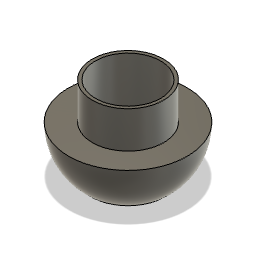
postreh_zarovka_v3 (Autodesk Fusion 360 design; units mm, degrees)
Autodesk Fusion 360 part; units mm, degrees
sketch "Sketch1" plane through (0, 0, 0) normal (0, 1, 0) x (1, 0, 0)
  circle A0 centre (0, 0) radius 25
  line L0 (23.097, 9.5671) -> (9.5671, 23.097)
  line L1 (9.5671, 23.097) -> (-9.5671, 23.097)
  line L2 (-9.5671, 23.097) -> (-23.097, 9.5671)
  line L3 (-23.097, 9.5671) -> (-23.097, -9.5671)
  line L4 (-23.097, -9.5671) -> (-9.5671, -23.097)
  line L5 (-9.5671, -23.097) -> (9.5671, -23.097)
  line L6 (9.5671, -23.097) -> (23.097, -9.5671)
  line L7 (23.097, -9.5671) -> (23.097, 9.5671)
  circle A1 centre (0, 0) radius 14
  line L8 (-5.25, 23.497) -> (5.25, 23.497)
  line L9 (5.25, 23.497) -> (5.25, 22.697)
  line L10 (5.25, 22.697) -> (-5.25, 22.697)
  line L11 (-5.25, 22.697) -> (-5.25, 23.497)
  line L12 (-5.25, 23.497) -> (5.25, 22.697) construction
  line L13 (5.25, 23.497) -> (-5.25, 22.697) construction
  line L14 (4.25, 25.2724) -> (-4.25, 25.2724)
  line L15 (-4.25, 25.2724) -> (-4.25, 21.7216)
  line L16 (-4.25, 21.7216) -> (4.25, 21.7216)
  line L17 (4.25, 21.7216) -> (4.25, 25.2724)
  line L18 (4.25, 25.2724) -> (-4.25, 21.7216) construction
  line L19 (-4.25, 25.2724) -> (4.25, 21.7216) construction
  line L20 (-12.3369, 19.7615) -> (-19.7615, 12.3369)
  line L21 (-12.9026, 20.3272) -> (-12.3369, 19.7615)
  line L22 (-20.3272, 12.9026) -> (-12.9026, 20.3272)
  line L23 (-12.3543, 18.3647) -> (-14.8651, 20.8755)
  line L24 (-18.3647, 12.3543) -> (-12.3543, 18.3647)
  line L25 (-20.8755, 14.8651) -> (-18.3647, 12.3543)
  line L26 (-19.7615, 12.3369) -> (-20.3272, 12.9026)
  line L27 (-14.8651, 20.8755) -> (-20.8755, 14.8651)
  line L28 (-22.697, 5.25) -> (-22.697, -5.25)
  line L29 (-23.497, 5.25) -> (-22.697, 5.25)
  line L30 (-23.497, -5.25) -> (-23.497, 5.25)
  line L31 (-21.7216, 4.25) -> (-25.2724, 4.25)
  line L32 (-21.7216, -4.25) -> (-21.7216, 4.25)
  line L33 (-25.2724, -4.25) -> (-21.7216, -4.25)
  line L34 (-22.697, -5.25) -> (-23.497, -5.25)
  line L35 (-25.2724, 4.25) -> (-25.2724, -4.25)
  line L36 (-19.7615, -12.3369) -> (-12.3369, -19.7615)
  line L37 (-20.3272, -12.9026) -> (-19.7615, -12.3369)
  line L38 (-12.9026, -20.3272) -> (-20.3272, -12.9026)
  line L39 (-18.3647, -12.3543) -> (-20.8755, -14.8651)
  line L40 (-12.3543, -18.3647) -> (-18.3647, -12.3543)
  line L41 (-14.8651, -20.8755) -> (-12.3543, -18.3647)
  line L42 (-12.3369, -19.7615) -> (-12.9026, -20.3272)
  line L43 (-20.8755, -14.8651) -> (-14.8651, -20.8755)
  line L44 (-5.25, -22.697) -> (5.25, -22.697)
  line L45 (-5.25, -23.497) -> (-5.25, -22.697)
  line L46 (5.25, -23.497) -> (-5.25, -23.497)
  line L47 (-4.25, -21.7216) -> (-4.25, -25.2724)
  line L48 (4.25, -21.7216) -> (-4.25, -21.7216)
  line L49 (4.25, -25.2724) -> (4.25, -21.7216)
  line L50 (5.25, -22.697) -> (5.25, -23.497)
  line L51 (-4.25, -25.2724) -> (4.25, -25.2724)
  line L52 (12.3369, -19.7615) -> (19.7615, -12.3369)
  line L53 (12.9026, -20.3272) -> (12.3369, -19.7615)
  line L54 (20.3272, -12.9026) -> (12.9026, -20.3272)
  line L55 (12.3543, -18.3647) -> (14.8651, -20.8755)
  line L56 (18.3647, -12.3543) -> (12.3543, -18.3647)
  line L57 (20.8755, -14.8651) -> (18.3647, -12.3543)
  line L58 (19.7615, -12.3369) -> (20.3272, -12.9026)
  line L59 (14.8651, -20.8755) -> (20.8755, -14.8651)
  line L60 (22.697, -5.25) -> (22.697, 5.25)
  line L61 (23.497, -5.25) -> (22.697, -5.25)
  line L62 (23.497, 5.25) -> (23.497, -5.25)
  line L63 (21.7216, -4.25) -> (25.2724, -4.25)
  line L64 (21.7216, 4.25) -> (21.7216, -4.25)
  line L65 (25.2724, 4.25) -> (21.7216, 4.25)
  line L66 (22.697, 5.25) -> (23.497, 5.25)
  line L67 (25.2724, -4.25) -> (25.2724, 4.25)
  line L68 (19.7615, 12.3369) -> (12.3369, 19.7615)
  line L69 (20.3272, 12.9026) -> (19.7615, 12.3369)
  line L70 (12.9026, 20.3272) -> (20.3272, 12.9026)
  line L71 (18.3647, 12.3543) -> (20.8755, 14.8651)
  line L72 (12.3543, 18.3647) -> (18.3647, 12.3543)
  line L73 (14.8651, 20.8755) -> (12.3543, 18.3647)
  line L74 (12.3369, 19.7615) -> (12.9026, 20.3272)
  line L75 (20.8755, 14.8651) -> (14.8651, 20.8755)
  point P0 (0, 23.097)
  point P1 (0, 23.497)
  dimension "d1" = 50
  dimension "d2" = 28
  dimension "d3" = 10.5
  dimension "d4" = 0.8
  dimension "d5" = 8.5
  dimension "d7" = 360
  constraint coincident A0.centre A1.centre
  constraint coincident A0 L0.start
  constraint concentric A0 A1
  constraint horizontal L8
  constraint perpendicular L8 L9
  constraint parallel L8 L10
  constraint parallel L9 L11
  constraint coincident L12 P0
  constraint coincident L13 P0
  constraint midpoint L1 P0
  constraint horizontal L14
  constraint perpendicular L14 L15
  constraint parallel L14 L16
  constraint parallel L15 L17
  constraint coincident L18 P1
  constraint coincident L19 P1
  constraint midpoint L8 P1
  measures "d1" diameter of A0
  measures "d2" diameter of A1
  measures "d3" distance of L9.end L10.end
  measures "d4" distance of L8.end L9.end
  measures "d5" distance of L15.end L16.end
extrude "Extrude1" add sketch "Sketch1" along normal blind 105 contours A0 L7 L62 L65 L66 | A0 L7 L61 L62 L63 | A0 L0 L69 L70 L71 | L0 L1 L2 L3 L4 L5 L6 L7 L9 L10 L11 L15 L16 L17 L20 L21 L23 L24 L25 L26 L28 L29 L31 L32 L33 L34 L36 L37 L39 L40 L41 L42 L44 L45 L47 L48 L49 L50 L52 L53 L55 L56 L57 L58 L60 L61 L63 L64 L65 L66 L68 L69 L71 L72 L73 L74 | A0 L6 L54 L57 L58 | A0 L0 L70 L73 L74 | L60 L63 L64 L65 | A0 L6 L53 L54 L55 | A0 L1 L8 L9 L17 | L68 L71 L72 L73 | A0 L5 L46 L49 L50 | L52 L55 L56 L57 | A0 L1 L8 L11 L15 | A0 L5 L45 L46 L47 | A0 L2 L21 L22 L23 | L10 L15 L16 L17 | A0 L4 L38 L41 L42 | L44 L47 L48 L49 | A0 L2 L22 L25 L26 | A0 L4 L37 L38 L39 | A0 L3 L29 L30 L31 | L20 L23 L24 L25 | A0 L3 L30 L33 L34 | L36 L39 L40 L41 | L28 L31 L32 L33 makes body 1
sketch "Sketch2" plane through (0, 0, 0) normal (0, 1, 0) x (1, 0, 0)
  circle A0 centre (91.4073, -5.9758) radius 17.5
  circle A1 centre (75.1447, -64.4139) radius 16.25
  dimension "d10" = 35
  dimension "d11" = 32.5
  measures "d10" diameter of A0
  measures "d11" diameter of A1
sketch "Sketch3" plane through (0, 105, 0) normal (0, 1, 0) x (-1, 0, 0)
  circle A0 centre (0, 0) radius 14
  line L0 (-19.6201, -13.6097) -> (-20.3272, -12.9026)
  line L1 (-20.3272, -12.9026) -> (-19.7615, -12.3369)
  line L2 (-19.7615, -12.3369) -> (-12.3369, -19.7615)
  line L3 (-12.3369, -19.7615) -> (-12.9026, -20.3272)
  line L4 (-12.9026, -20.3272) -> (-13.6097, -19.6201)
  line L5 (-13.6097, -19.6201) -> (-14.4152, -20.4256)
  arc A1 (-14.4152, -20.4256) -> (-4.25, -24.6361) centre (0, 0) ccw
  line L6 (-4.25, -24.6361) -> (-4.25, -23.497)
  line L7 (-4.25, -23.497) -> (-5.25, -23.497)
  line L8 (-5.25, -23.497) -> (-5.25, -22.697)
  line L9 (-5.25, -22.697) -> (5.25, -22.697)
  line L10 (5.25, -22.697) -> (5.25, -23.497)
  line L11 (5.25, -23.497) -> (4.25, -23.497)
  line L12 (4.25, -23.497) -> (4.25, -24.6361)
  arc A2 (4.25, -24.6361) -> (14.4152, -20.4256) centre (0, 0) ccw
  line L13 (14.4152, -20.4256) -> (13.6097, -19.6201)
  line L14 (13.6097, -19.6201) -> (12.9026, -20.3272)
  line L15 (12.9026, -20.3272) -> (12.3369, -19.7615)
  line L16 (12.3369, -19.7615) -> (19.7615, -12.3369)
  line L17 (19.7615, -12.3369) -> (20.3272, -12.9026)
  line L18 (20.3272, -12.9026) -> (19.6201, -13.6097)
  line L19 (19.6201, -13.6097) -> (20.4256, -14.4152)
  arc A3 (20.4256, -14.4152) -> (24.6361, -4.25) centre (0, 0) ccw
  line L20 (24.6361, -4.25) -> (23.497, -4.25)
  line L21 (23.497, -4.25) -> (23.497, -5.25)
  line L22 (23.497, -5.25) -> (22.697, -5.25)
  line L23 (22.697, -5.25) -> (22.697, 5.25)
  line L24 (22.697, 5.25) -> (23.497, 5.25)
  line L25 (23.497, 5.25) -> (23.497, 4.25)
  line L26 (23.497, 4.25) -> (24.6361, 4.25)
  arc A4 (24.6361, 4.25) -> (20.4256, 14.4152) centre (0, 0) ccw
  line L27 (20.4256, 14.4152) -> (19.6201, 13.6097)
  line L28 (19.6201, 13.6097) -> (20.3272, 12.9026)
  line L29 (20.3272, 12.9026) -> (19.7615, 12.3369)
  line L30 (19.7615, 12.3369) -> (12.3369, 19.7615)
  line L31 (12.3369, 19.7615) -> (12.9026, 20.3272)
  line L32 (12.9026, 20.3272) -> (13.6097, 19.6201)
  line L33 (13.6097, 19.6201) -> (14.4152, 20.4256)
  arc A5 (14.4152, 20.4256) -> (4.25, 24.6361) centre (0, 0) ccw
  line L34 (4.25, 24.6361) -> (4.25, 23.497)
  line L35 (4.25, 23.497) -> (5.25, 23.497)
  line L36 (5.25, 23.497) -> (5.25, 22.697)
  line L37 (5.25, 22.697) -> (-5.25, 22.697)
  line L38 (-5.25, 22.697) -> (-5.25, 23.497)
  line L39 (-5.25, 23.497) -> (-4.25, 23.497)
  line L40 (-4.25, 23.497) -> (-4.25, 24.6361)
  arc A6 (-4.25, 24.6361) -> (-14.4152, 20.4256) centre (0, 0) ccw
  line L41 (-14.4152, 20.4256) -> (-13.6097, 19.6201)
  line L42 (-13.6097, 19.6201) -> (-12.9026, 20.3272)
  line L43 (-12.9026, 20.3272) -> (-12.3369, 19.7615)
  line L44 (-12.3369, 19.7615) -> (-19.7615, 12.3369)
  line L45 (-19.7615, 12.3369) -> (-20.3272, 12.9026)
  line L46 (-20.3272, 12.9026) -> (-19.6201, 13.6097)
  line L47 (-19.6201, 13.6097) -> (-20.4256, 14.4152)
  arc A7 (-20.4256, 14.4152) -> (-24.6361, 4.25) centre (0, 0) ccw
  line L48 (-24.6361, 4.25) -> (-23.497, 4.25)
  line L49 (-23.497, 4.25) -> (-23.497, 5.25)
  line L50 (-23.497, 5.25) -> (-22.697, 5.25)
  line L51 (-22.697, 5.25) -> (-22.697, -5.25)
  line L52 (-22.697, -5.25) -> (-23.497, -5.25)
  line L53 (-23.497, -5.25) -> (-23.497, -4.25)
  line L54 (-23.497, -4.25) -> (-24.6361, -4.25)
  arc A8 (-24.6361, -4.25) -> (-20.4256, -14.4152) centre (0, 0) ccw
  line L55 (-20.4256, -14.4152) -> (-19.6201, -13.6097)
  circle A9 centre (0, 0) radius 17.5
  dimension "d16" = 35
  constraint concentric A0 A9
  measures "d16" diameter of A9
extrude "Extrude3" add sketch "Sketch3" along normal blind 12 contours A0 | A9 bodies 1
chamfer "Chamfer1" distance 4 angle 45 1 edges at (-13.0526, 105, -5.0626) on bodies 1
extrude "Extrude4" cut 1 faces at (-2.8212, 105, -0.9825) along direction (0, 1, 0) blind 44 on bodies 1 bodies 1
ref_plane "WorkPlane3" through (0, 117, 0) normal (0, 1, 0) x (-1, 0, 0)
ref_plane "WorkPlane4" through (0, 114, 0) normal (0, 1, 0) x (-1, 0, 0)
ref_plane "WorkPlane5" through (0, 111, 0) normal (0, 1, 0) x (-1, 0, 0)
thread "Thread3" "ANSI Unified Screw Threads 1.375 1 3/8-8 UN 3A" major diameter 34.7345 minor diameter 31.1455 pitch 3.175 angle 60 modelled right hand crest width 0.4671 on face at (-17.4433, 113, -1.4082) crest through (-17.3672, 104.2062, 0) on bodies 1
sketch "Sketch4" plane through (0, 105, 0) normal (0, 1, 0) x (-1, 0, 0)
  arc A0 (7.7444, 15.545) -> (-7.7444, 15.545) centre (0, 0) ccw
  spline S0 degree 3 poles (7.7444, 15.545) (8.9942, 14.8417) (10.1519, 13.9862) (12.214, 12.0191) (13.1134, 10.9184) (15.0227, 7.8711) (15.8119, 5.8174) (16.5433, 1.5647) (16.4948, -0.5901) (15.5763, -4.7155) (14.7314, -6.6497) (12.3661, -10.0449) (10.8824, -11.4824) (9.1629, -12.5917) knots -3.386882 -3.386882 -3.386882 -3.386882 -2.957534 -2.957534 -2.533537 -2.533537 -1.880654 -1.880654 -1.240767 -1.240767 -0.613881 -0.613881 0 0 0 0
  arc A1 (-9.1629, -12.5917) -> (9.1629, -12.5917) centre (0, 0) ccw
  spline S1 degree 3 poles (-9.1629, -12.5917) (-10.2571, -11.8858) (-11.2583, -11.0453) (-13.0433, -9.1242) (-13.8169, -8.0481) (-15.4568, -5.0428) (-16.0901, -3.016) (-16.5572, 1.21) (-16.3698, 3.3701) (-15.173, 7.5422) (-14.1591, 9.5092) (-11.4129, 12.984) (-9.6941, 14.4478) (-7.7444, 15.545) knots -3.394641 -3.394641 -3.394641 -3.394641 -3.003225 -3.003225 -2.606447 -2.606447 -1.974373 -1.974373 -1.32927 -1.32927 -0.671144 -0.671144 0 0 0 0
  line L0 (-19.6201, -13.6097) -> (-20.3272, -12.9026)
  line L1 (-20.3272, -12.9026) -> (-19.7615, -12.3369)
  line L2 (-19.7615, -12.3369) -> (-12.3369, -19.7615)
  line L3 (-12.3369, -19.7615) -> (-12.9026, -20.3272)
  line L4 (-12.9026, -20.3272) -> (-13.6097, -19.6201)
  line L5 (-13.6097, -19.6201) -> (-14.4152, -20.4256)
  arc A2 (-14.4152, -20.4256) -> (-4.25, -24.6361) centre (0, 0) ccw
  line L6 (-4.25, -24.6361) -> (-4.25, -23.497)
  line L7 (-4.25, -23.497) -> (-5.25, -23.497)
  line L8 (-5.25, -23.497) -> (-5.25, -22.697)
  line L9 (-5.25, -22.697) -> (5.25, -22.697)
  line L10 (5.25, -22.697) -> (5.25, -23.497)
  line L11 (5.25, -23.497) -> (4.25, -23.497)
  line L12 (4.25, -23.497) -> (4.25, -24.6361)
  arc A3 (4.25, -24.6361) -> (14.4152, -20.4256) centre (0, 0) ccw
  line L13 (14.4152, -20.4256) -> (13.6097, -19.6201)
  line L14 (13.6097, -19.6201) -> (12.9026, -20.3272)
  line L15 (12.9026, -20.3272) -> (12.3369, -19.7615)
  line L16 (12.3369, -19.7615) -> (19.7615, -12.3369)
  line L17 (19.7615, -12.3369) -> (20.3272, -12.9026)
  line L18 (20.3272, -12.9026) -> (19.6201, -13.6097)
  line L19 (19.6201, -13.6097) -> (20.4256, -14.4152)
  arc A4 (20.4256, -14.4152) -> (24.6361, -4.25) centre (0, 0) ccw
  line L20 (24.6361, -4.25) -> (23.497, -4.25)
  line L21 (23.497, -4.25) -> (23.497, -5.25)
  line L22 (23.497, -5.25) -> (22.697, -5.25)
  line L23 (22.697, -5.25) -> (22.697, 5.25)
  line L24 (22.697, 5.25) -> (23.497, 5.25)
  line L25 (23.497, 5.25) -> (23.497, 4.25)
  line L26 (23.497, 4.25) -> (24.6361, 4.25)
  arc A5 (24.6361, 4.25) -> (20.4256, 14.4152) centre (0, 0) ccw
  line L27 (20.4256, 14.4152) -> (19.6201, 13.6097)
  line L28 (19.6201, 13.6097) -> (20.3272, 12.9026)
  line L29 (20.3272, 12.9026) -> (19.7615, 12.3369)
  line L30 (19.7615, 12.3369) -> (12.3369, 19.7615)
  line L31 (12.3369, 19.7615) -> (12.9026, 20.3272)
  line L32 (12.9026, 20.3272) -> (13.6097, 19.6201)
  line L33 (13.6097, 19.6201) -> (14.4152, 20.4256)
  arc A6 (14.4152, 20.4256) -> (4.25, 24.6361) centre (0, 0) ccw
  line L34 (4.25, 24.6361) -> (4.25, 23.497)
  line L35 (4.25, 23.497) -> (5.25, 23.497)
  line L36 (5.25, 23.497) -> (5.25, 22.697)
  line L37 (5.25, 22.697) -> (-5.25, 22.697)
  line L38 (-5.25, 22.697) -> (-5.25, 23.497)
  line L39 (-5.25, 23.497) -> (-4.25, 23.497)
  line L40 (-4.25, 23.497) -> (-4.25, 24.6361)
  arc A7 (-4.25, 24.6361) -> (-14.4152, 20.4256) centre (0, 0) ccw
  line L41 (-14.4152, 20.4256) -> (-13.6097, 19.6201)
  line L42 (-13.6097, 19.6201) -> (-12.9026, 20.3272)
  line L43 (-12.9026, 20.3272) -> (-12.3369, 19.7615)
  line L44 (-12.3369, 19.7615) -> (-19.7615, 12.3369)
  line L45 (-19.7615, 12.3369) -> (-20.3272, 12.9026)
  line L46 (-20.3272, 12.9026) -> (-19.6201, 13.6097)
  line L47 (-19.6201, 13.6097) -> (-20.4256, 14.4152)
  arc A8 (-20.4256, 14.4152) -> (-24.6361, 4.25) centre (0, 0) ccw
  line L48 (-24.6361, 4.25) -> (-23.497, 4.25)
  line L49 (-23.497, 4.25) -> (-23.497, 5.25)
  line L50 (-23.497, 5.25) -> (-22.697, 5.25)
  line L51 (-22.697, 5.25) -> (-22.697, -5.25)
  line L52 (-22.697, -5.25) -> (-23.497, -5.25)
  line L53 (-23.497, -5.25) -> (-23.497, -4.25)
  line L54 (-23.497, -4.25) -> (-24.6361, -4.25)
  arc A9 (-24.6361, -4.25) -> (-20.4256, -14.4152) centre (0, 0) ccw
  line L55 (-20.4256, -14.4152) -> (-19.6201, -13.6097)
  circle A10 centre (0, 0) radius 27.4518
  circle A11 centre (0, 0) radius 18
  line L56 (19.7615, -12.3369) -> (12.3369, -19.7615)
  line L57 (5.25, -22.697) -> (12.3369, -19.7615)
  line L58 (5.25, -22.697) -> (-5.25, -22.697)
  line L59 (-5.25, -22.697) -> (-12.3369, -19.7615)
  line L60 (-19.7615, -12.3369) -> (-12.3369, -19.7615)
  line L61 (-19.7615, -12.3369) -> (-22.697, -5.25)
  line L62 (-22.697, -5.25) -> (-22.697, 5.25)
  line L63 (-22.697, 5.25) -> (-19.7615, 12.3369)
  line L64 (-19.7615, 12.3369) -> (-12.3369, 19.7615)
  line L65 (-12.3369, 19.7615) -> (-5.25, 22.697)
  line L66 (-5.25, 22.697) -> (5.25, 22.697)
  line L67 (5.25, 22.697) -> (12.3369, 19.7615)
  line L68 (12.3369, 19.7615) -> (19.7615, 12.3369)
  line L69 (19.7615, 12.3369) -> (22.697, 5.25)
  line L70 (22.697, 5.25) -> (22.697, -5.25)
  line L71 (22.697, -5.25) -> (19.7615, -12.3369)
  dimension "d25" = 36
  constraint concentric A0 A10
  constraint concentric A0 A11
  constraint coincident L16.end L17.start
  constraint coincident L15.end L16.start
  constraint coincident L9.end L10.start
  constraint coincident L8.end L9.start
  constraint coincident L2.end L3.start
  constraint coincident L1.end L2.start
  constraint coincident L51.end L52.start
  constraint coincident L50.end L51.start
  constraint coincident L44.end L45.start
  constraint coincident L43.end L44.start
  constraint coincident L37.end L38.start
  constraint coincident L36.end L37.start
  constraint coincident L30.end L31.start
  constraint coincident L29.end L30.start
  constraint coincident L23.end L24.start
  constraint coincident L22.end L23.start
  measures "d25" diameter of A11
extrude "Extrude5" cut sketch "Sketch4" against normal blind 8 contours L0 L1 L52 L53 L54 A9 L55 L61 | L3 L4 L5 A2 L6 L7 L8 L59 | L45 L46 L47 A8 L48 L49 L50 L63 | L10 L11 L12 A3 L13 L14 L15 L57 | L38 L39 L40 A7 L41 L42 L43 L65 | L17 L18 L19 A4 L20 L21 L22 L71 | L31 L32 L33 A6 L34 L35 L36 L67 | L24 L25 L26 A5 L27 L28 L29 L69 bodies 1
sketch "Sketch5" plane through (21.2292, 0, 8.7934) normal (0.92388, 0, 0.382683) x (0.382683, 0, -0.92388)
  line L0 (3.8354, 105) -> (-3.8354, 105)
  line L1 (-3.8354, 105) -> (-3.8354, 97)
  line L2 (-3.8354, 97) -> (3.8354, 97)
  line L3 (3.8354, 97) -> (3.8354, 105)
  line L4 (-3.8354, 105) -> (3.8354, 105)
  line L5 (3.8354, 105) -> (3.8354, 97.329)
  line L6 (3.8354, 97.329) -> (-3.8354, 97.329)
  line L7 (-3.8354, 97.329) -> (-3.8354, 105)
  circle A0 centre (0, 101) radius 2.5
  dimension "d28" = 7.671
  dimension "d29" = 5
  constraint horizontal L4
  constraint vertical L5
  constraint horizontal L6
  constraint vertical L7
  constraint coincident L0.end L1.start
  measures "d28" distance of L0.end L6.end
  measures "d29" diameter of A0
extrude "Extrude6" cut sketch "Sketch5" against normal blind 52 contours A0 bodies 1
sketch "Sketch6" plane through (21.2292, 0, -8.7934) normal (0.92388, 0, -0.382683) x (-0.382683, 0, -0.92388)
  line L0 (3.8354, 105) -> (-3.8354, 105)
  line L1 (-3.8354, 105) -> (-3.8354, 97)
  line L2 (-3.8354, 97) -> (3.8354, 97)
  line L3 (3.8354, 97) -> (3.8354, 105)
  line L4 (-3.8354, 105) -> (3.8354, 105)
  line L5 (3.8354, 105) -> (3.8354, 97.329)
  line L6 (3.8354, 97.329) -> (-3.8354, 97.329)
  line L7 (-3.8354, 97.329) -> (-3.8354, 105)
  circle A0 centre (0, 101.1645) radius 2.5
  dimension "d32" = 7.671
  dimension "d33" = 5
  constraint horizontal L4
  constraint vertical L5
  constraint horizontal L6
  constraint vertical L7
  constraint coincident L0.end L1.start
  measures "d32" distance of L0.end L6.end
  measures "d33" diameter of A0
extrude "Extrude7" cut sketch "Sketch6" against normal blind 103 contours A0 bodies 1
sketch "Sketch7" plane through (8.7934, 0, -21.2292) normal (0.382683, 0, -0.92388) x (-0.92388, 0, -0.382683)
  line L0 (3.8354, 105) -> (-3.8354, 105)
  line L1 (-3.8354, 105) -> (-3.8354, 97)
  line L2 (-3.8354, 97) -> (3.8354, 97)
  line L3 (3.8354, 97) -> (3.8354, 105)
  line L4 (-3.8354, 105) -> (3.8354, 105)
  line L5 (3.8354, 105) -> (3.8354, 97.329)
  line L6 (3.8354, 97.329) -> (-3.8354, 97.329)
  line L7 (-3.8354, 97.329) -> (-3.8354, 105)
  circle A0 centre (0, 101) radius 2.5
  dimension "d36" = 7.671
  dimension "d37" = 5
  constraint horizontal L4
  constraint vertical L5
  constraint horizontal L6
  constraint vertical L7
  constraint coincident L0.end L1.start
  measures "d36" distance of L0.end L6.end
  measures "d37" diameter of A0
extrude "Extrude8" cut sketch "Sketch7" against normal blind 84 contours A0 bodies 1
sketch "Sketch8" plane through (-8.7934, 0, -21.2292) normal (-0.382683, 0, -0.92388) x (-0.92388, 0, 0.382683)
  line L0 (3.8354, 105) -> (-3.8354, 105)
  line L1 (-3.8354, 105) -> (-3.8354, 97)
  line L2 (-3.8354, 97) -> (3.8354, 97)
  line L3 (3.8354, 97) -> (3.8354, 105)
  line L4 (-3.8354, 105) -> (3.8354, 105)
  line L5 (3.8354, 105) -> (3.8354, 97.329)
  line L6 (3.8354, 97.329) -> (-3.8354, 97.329)
  line L7 (-3.8354, 97.329) -> (-3.8354, 105)
  circle A0 centre (0, 101.1645) radius 2.5
  dimension "d40" = 7.671
  dimension "d41" = 5
  constraint horizontal L4
  constraint vertical L5
  constraint horizontal L6
  constraint vertical L7
  constraint coincident L0.end L1.start
  measures "d40" distance of L0.end L6.end
  measures "d41" diameter of A0
extrude "Extrude9" cut sketch "Sketch8" against normal blind 69 contours A0 bodies 1
sphere "SpherePrimitive1" add diameter 45.2 placed x (1, 0, 0) y (0, 0, -1) z (0, 1, 0) at (0, 0, 0) separate body makes body 2
ref_plane "WorkPlane6" through (0, 0, 0) normal (0, -1, 0) x (-1, 0, 0)
split "Split1" by plane through (0, 0, 0) normal (0, -1, 0) bodies 2 makes body 3 at (-11.2033, -2.9499, 19.4047)
delete_body "RemoveBody1" bodies 2
sketch "Sketch10" plane through (0, 0, 0) normal (0, -1, 0) x (1, 0, 0)
  circle A0 centre (0, 0) radius 14
  line L0 (20.3272, -12.9026) -> (19.6201, -13.6097)
  line L1 (19.6201, -13.6097) -> (20.4256, -14.4152)
  arc A1 (20.4256, -14.4152) -> (24.6361, -4.25) centre (0, 0) ccw
  line L2 (24.6361, -4.25) -> (23.497, -4.25)
  line L3 (23.497, -4.25) -> (23.497, -5.25)
  line L4 (23.497, -5.25) -> (22.697, -5.25)
  line L5 (22.697, -5.25) -> (22.697, 5.25)
  line L6 (22.697, 5.25) -> (23.497, 5.25)
  line L7 (23.497, 5.25) -> (23.497, 4.25)
  line L8 (23.497, 4.25) -> (24.6361, 4.25)
  arc A2 (24.6361, 4.25) -> (20.4256, 14.4152) centre (0, 0) ccw
  line L9 (20.4256, 14.4152) -> (19.6201, 13.6097)
  line L10 (19.6201, 13.6097) -> (20.3272, 12.9026)
  line L11 (20.3272, 12.9026) -> (19.7615, 12.3369)
  line L12 (19.7615, 12.3369) -> (12.3369, 19.7615)
  line L13 (12.3369, 19.7615) -> (12.9026, 20.3272)
  line L14 (12.9026, 20.3272) -> (13.6097, 19.6201)
  line L15 (13.6097, 19.6201) -> (14.4152, 20.4256)
  arc A3 (14.4152, 20.4256) -> (4.25, 24.6361) centre (0, 0) ccw
  line L16 (4.25, 24.6361) -> (4.25, 23.497)
  line L17 (4.25, 23.497) -> (5.25, 23.497)
  line L18 (5.25, 23.497) -> (5.25, 22.697)
  line L19 (5.25, 22.697) -> (-5.25, 22.697)
  line L20 (-5.25, 22.697) -> (-5.25, 23.497)
  line L21 (-5.25, 23.497) -> (-4.25, 23.497)
  line L22 (-4.25, 23.497) -> (-4.25, 24.6361)
  arc A4 (-4.25, 24.6361) -> (-14.4152, 20.4256) centre (0, 0) ccw
  line L23 (-14.4152, 20.4256) -> (-13.6097, 19.6201)
  line L24 (-13.6097, 19.6201) -> (-12.9026, 20.3272)
  line L25 (-12.9026, 20.3272) -> (-12.3369, 19.7615)
  line L26 (-12.3369, 19.7615) -> (-19.7615, 12.3369)
  line L27 (-19.7615, 12.3369) -> (-20.3272, 12.9026)
  line L28 (-20.3272, 12.9026) -> (-19.6201, 13.6097)
  line L29 (-19.6201, 13.6097) -> (-20.4256, 14.4152)
  arc A5 (-20.4256, 14.4152) -> (-24.6361, 4.25) centre (0, 0) ccw
  line L30 (-24.6361, 4.25) -> (-23.497, 4.25)
  line L31 (-23.497, 4.25) -> (-23.497, 5.25)
  line L32 (-23.497, 5.25) -> (-22.697, 5.25)
  line L33 (-22.697, 5.25) -> (-22.697, -5.25)
  line L34 (-22.697, -5.25) -> (-23.497, -5.25)
  line L35 (-23.497, -5.25) -> (-23.497, -4.25)
  line L36 (-23.497, -4.25) -> (-24.6361, -4.25)
  arc A6 (-24.6361, -4.25) -> (-20.4256, -14.4152) centre (0, 0) ccw
  line L37 (-20.4256, -14.4152) -> (-19.6201, -13.6097)
  line L38 (-19.6201, -13.6097) -> (-20.3272, -12.9026)
  line L39 (-20.3272, -12.9026) -> (-19.7615, -12.3369)
  line L40 (-19.7615, -12.3369) -> (-12.3369, -19.7615)
  line L41 (-12.3369, -19.7615) -> (-12.9026, -20.3272)
  line L42 (-12.9026, -20.3272) -> (-13.6097, -19.6201)
  line L43 (-13.6097, -19.6201) -> (-14.4152, -20.4256)
  arc A7 (-14.4152, -20.4256) -> (-4.25, -24.6361) centre (0, 0) ccw
  line L44 (-4.25, -24.6361) -> (-4.25, -23.497)
  line L45 (-4.25, -23.497) -> (-5.25, -23.497)
  line L46 (-5.25, -23.497) -> (-5.25, -22.697)
  line L47 (-5.25, -22.697) -> (5.25, -22.697)
  line L48 (5.25, -22.697) -> (5.25, -23.497)
  line L49 (5.25, -23.497) -> (4.25, -23.497)
  line L50 (4.25, -23.497) -> (4.25, -24.6361)
  arc A8 (4.25, -24.6361) -> (14.4152, -20.4256) centre (0, 0) ccw
  line L51 (14.4152, -20.4256) -> (13.6097, -19.6201)
  line L52 (13.6097, -19.6201) -> (12.9026, -20.3272)
  line L53 (12.9026, -20.3272) -> (12.3369, -19.7615)
  line L54 (12.3369, -19.7615) -> (19.7615, -12.3369)
  line L55 (19.7615, -12.3369) -> (20.3272, -12.9026)
  circle A9 centre (0, 0) radius 13.6
  circle A10 centre (0, 0) radius 12.4
  dimension "d46" = 27.2
  dimension "d47" = 24.8
  constraint concentric A0 A9
  constraint coincident A0.centre A1.centre
  measures "d46" diameter of A9
  measures "d47" diameter of A10
extrude "Extrude10" add sketch "Sketch10" against normal blind 14 separate body contours A9 makes body 4
sketch "Sketch11" plane through (0, 0, 0) normal (0, -1, 0) x (1, 0, 0)
  circle A0 centre (0, 0) radius 12.4
  circle A1 centre (0, 0) radius 13.6
extrude "Extrude11" cut sketch "Sketch11" along normal blind 55 contours A0 bodies 3
fillet "Fillet1" radius 1 1 edges at (-11.5609, -18.8944, 4.484) on bodies 3
combine "Combine1" operation add target body 3 tool bodies 4
hidden bodies 1
equation "d5 = 10.500 mm - 2 mm"
equation "d46 = 28.000 mm - 0.8 mm"
equation "d47 = 27.200 mm - ( 1.2 * 2 ) * 1 mm"
named bodies: "spunt"
